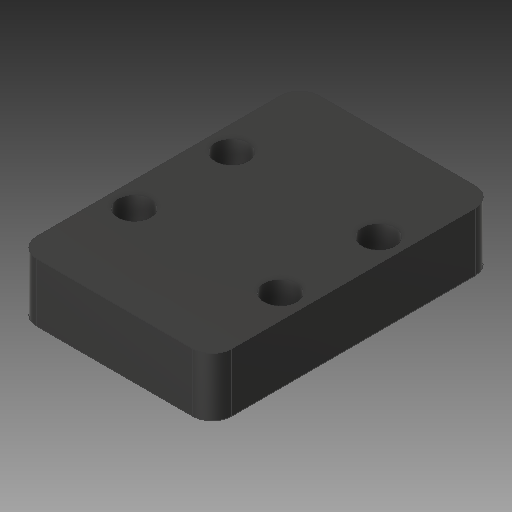
# Autodesk Inventor part: 6mm XY Packer Block
Saved by Autodesk Inventor 2019 (Build 230136000, 136)
## iProperties
Created: 2018-10-20
Part Number: 6mm XY Packer Block
Material: ABS Plastic
Document SubType Name: Modeling
Designer: Ax
Density: 1.06 g/cm^3
Appearance: Smooth - Black
Mass: 3.43599 g
Surface Area: 19.0425 cm^2
Volume: 3.2415 cm^3
Author: Ax
Autodesk Inventor part; units mm, degrees
ref_plane "YZ Plane" through (0, 0, 0) normal (1, 0, 0) x (0, 1, 0)
ref_plane "XZ Plane" through (0, 0, 0) normal (0, 1, 0) x (-1, 0, 0)
ref_plane "XY Plane" through (0, 0, 0) normal (0, 0, 1) x (1, 0, 0)
sketch "Sketch1" plane through (0, 0, 0) normal (0, 1, 0) x (-1, 0, 0)
  line L0 (-10, 14.5) -> (10, 14.5)
  line L1 (10, 14.5) -> (10, -14.5)
  line L2 (10, -14.5) -> (-10, -14.5)
  line L3 (-10, -14.5) -> (-10, 14.5)
  line L4 (-10, 14.5) -> (10, -14.5) construction
  line L5 (10, 14.5) -> (-10, -14.5) construction
  line L6 (-7.5, 5) -> (7.5, 5) construction
  line L7 (7.5, 5) -> (7.5, -5) construction
  line L8 (7.5, -5) -> (-7.5, -5) construction
  line L9 (-7.5, -5) -> (-7.5, 5) construction
  line L10 (-7.5, 5) -> (7.5, -5) construction
  line L11 (7.5, 5) -> (-7.5, -5) construction
  circle A0 centre (7.5, -5) radius 1.7
  circle A1 centre (-7.5872, -5) radius 1.7
  circle A2 centre (-7.5, 5) radius 1.7
  circle A3 centre (7.5, 5) radius 1.7
  point P0 (0, 0)
  dimension "d0" = 29
  dimension "d1" = 20
  dimension "d2" = 15
  dimension "d3" = 10
  dimension "d4" = 3.4
  constraints: 24 end point, 4 centre point, 4 midpoint, 4 parallel, 3 coincident, 3 equal radius, 2 horizontal, 2 perpendicular
  measures "d0" distance of L0.end L1.end
  measures "d1" distance of L1.end L2.end
  measures "d2" distance of L7.end L8.end
  measures "d3" distance of L6.end L7.end
  measures "d4" diameter of A3
extrude "Extrusion1" add sketch "Sketch1" along normal blind 6
fillet "Fillet1" radius 2 4 edges at (10, 3, -14.5) (-10, 3, -14.5) (-10, 3, 14.5) (10, 3, 14.5)
body "Solid1"
